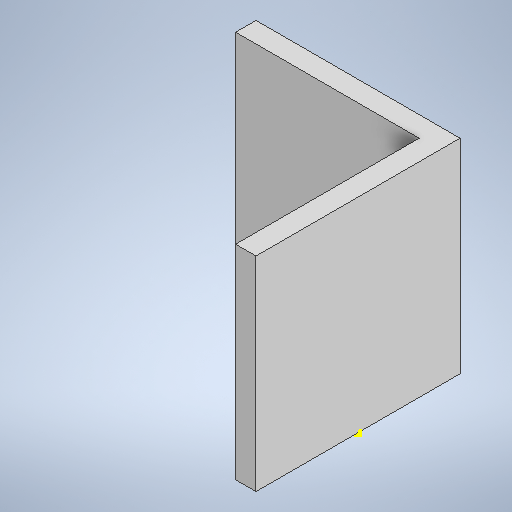
# Autodesk Inventor part: Soccer Goal Split
Saved by Autodesk Inventor 2026.1 (Build 301233000, 233)
## iProperties
Created: 2026-01-06
Part Number: Soccer Goal Split
Material: Generic
Document SubType Name: Modeling
Designer: User
Density: 1 g/cm^3
Appearance: Default
Author: User
Autodesk Inventor part; units mm, degrees
ref_plane "YZ Plane" through (0, 0, 0) normal (1, 0, 0) x (0, 1, 0)
ref_plane "XZ Plane" through (0, 0, 0) normal (0, 1, 0) x (-1, 0, 0)
ref_plane "XY Plane" through (0, 0, 0) normal (0, 0, 1) x (1, 0, 0)
sketch "Sketch1" plane through (0, 0, 0) normal (0, 1, 0) x (-1, 0, 0)
  line L0 (400, -50) -> (400, 50)
  line L1 (400, 50) -> (390, 50)
  line L2 (390, 50) -> (390, -40)
  line L3 (390, -40) -> (300, -40)
  line L4 (300, -40) -> (300, -50)
  line L5 (300, -50) -> (400, -50)
  line L6 (250, -50) -> (250, -40)
  line L7 (250, -40) -> (150, -40)
  line L8 (150, -40) -> (150, -50)
  line L9 (150, -50) -> (250, -50)
  line L10 (100, -50) -> (100, -40)
  line L11 (100, -40) -> (10, -40)
  line L12 (10, -40) -> (10, 50)
  line L13 (10, 50) -> (0, 50)
  line L14 (0, 50) -> (0, -50)
  line L15 (0, -50) -> (100, -50)
  point P0 (0, 0)
  dimension "d0" = 100
  dimension "d1" = 100
  dimension "d2" = 10
  dimension "d3" = 10
  dimension "d4" = 100
  dimension "d5" = 100
  dimension "d6" = 100
  dimension "d7" = 10
  dimension "d8" = 10
  dimension "d9" = 50
  dimension "d10" = 50
  dimension "d11" = 400
  dimension "d12" = 50
  dimension "d13" = 50
  constraints: 32 end point, 13 perpendicular, 4 point on line, 2 vertical
  measures "d0" distance of L0.start L0.end
  measures "d1" distance of L4.end L0.start
  measures "d2" distance of L0.end L1.end
  measures "d3" distance of L3.end L4.end
  measures "d4" distance of L8.end L6.start
  measures "d5" distance of L14.end L10.start
  measures "d6" distance of L13.end L14.end
  measures "d7" distance of L12.end L13.end
  measures "d8" distance of L10.start L10.end
  measures "d9" distance from line of L6.end L4
  measures "d10" distance between parallel lines of L10 L8
  measures "d11" distance from line of L0 point (0, 0)
  measures "d12" distance from line of point (0, 0) L5
  measures "d13" distance from line of point (0, 0) L13
extrude "Extrusion1" add sketch "Sketch1" along normal blind 100
sketch "Sketch2" plane through (0, 0, 0) normal (1, 0, 0) x (0, 1, 0)
  point P0 (0, 0)
sketch "Sketch3" plane through (0, 0, 50) normal (1, 0, 0) x (0, 0, -1)
  line L0 (92.5, 80) -> (97.5, 80)
  line L1 (97.5, 80) -> (97.5, 75)
  line L2 (97.5, 75) -> (92.5, 75)
  line L3 (92.5, 75) -> (92.5, 80)
  line L4 (97.5, 20) -> (92.5, 20)
  line L5 (92.5, 20) -> (92.5, 25)
  line L6 (92.5, 25) -> (97.5, 25)
  line L7 (97.5, 25) -> (97.5, 20)
  line L8 (0, 100) -> (100, 100) projected
  line L9 (100, 0) -> (100, 100) projected
  line L10 (0, 0) -> (100, 0) projected
  line L11 (92.5, 52.5) -> (97.5, 52.5)
  line L12 (97.5, 52.5) -> (97.5, 47.5)
  line L13 (97.5, 47.5) -> (92.5, 47.5)
  line L14 (92.5, 47.5) -> (92.5, 52.5)
  point P0 (50, 0)
  dimension "d16" = 20
  dimension "d17" = 5
  dimension "d18" = 5
  dimension "d19" = 2.5
  dimension "d20" = 20
  dimension "d21" = 5
  dimension "d22" = 5
  dimension "d24" = 7.5
  dimension "d25" = 5
  dimension "d26" = 5
  dimension "d27" = 2.5
  dimension "d28" = 22.5
  constraints: 24 end point, 6 parallel, 3 horizontal, 3 perpendicular
  measures "d16" distance between parallel lines of L8 L0
  measures "d17" distance of L1.end L2.end
  measures "d18" distance of L0.end L1.end
  measures "d19" distance between parallel lines of L9 L1
  measures "d20" distance between parallel lines of L10 L4
  measures "d21" distance of L6.end L4.start
  measures "d22" distance of L5.end L6.end
  measures "d24" distance between parallel lines of L9 L5
  measures "d25" distance of L13.end L11.start
  measures "d26" distance of L11.start L11.end
  measures "d27" distance between parallel lines of L9 L12
  measures "d28" distance between parallel lines of L2 L11
extrude "Extrusion2" cut sketch "Sketch3" against normal blind 320
sketch "Sketch4" plane through (0, 0, 50) normal (1, 0, 0) x (0, 0, -1)
  line L0 (97.5, 75) -> (92.5, 75) projected
  line L1 (97.5, 80) -> (97.5, 75) projected
  line L2 (92.5, 80) -> (97.5, 80) projected
  line L3 (92.5, 75) -> (92.5, 80) projected
  line L4 (97.5, 47.5) -> (92.5, 47.5) projected
  line L5 (97.5, 52.5) -> (97.5, 47.5) projected
  line L6 (92.5, 52.5) -> (97.5, 52.5) projected
  line L7 (92.5, 47.5) -> (92.5, 52.5) projected
  line L8 (92.5, 25) -> (97.5, 25) projected
  line L9 (92.5, 20) -> (92.5, 25) projected
  line L10 (97.5, 20) -> (92.5, 20) projected
  line L11 (97.5, 25) -> (97.5, 20) projected
  line L12 (92.5, 80) -> (97.5, 80)
  line L13 (97.5, 80) -> (97.5, 75)
  line L14 (97.5, 75) -> (92.5, 75)
  line L15 (92.5, 75) -> (92.5, 80)
  line L16 (92.5, 52.5) -> (97.5, 52.5)
  line L17 (97.5, 52.5) -> (97.5, 47.5)
  line L18 (97.5, 47.5) -> (92.5, 47.5)
  line L19 (92.5, 47.5) -> (92.5, 52.5)
  line L20 (92.5, 25) -> (97.5, 25)
  line L21 (97.5, 25) -> (97.5, 20)
  line L22 (97.5, 20) -> (92.5, 20)
  line L23 (92.5, 20) -> (92.5, 25)
  point P0 (50, 0)
  constraints: 24 end point, 6 parallel, 3 horizontal, 3 perpendicular
extrude "Extrusion3" add sketch "Sketch4" against normal blind 80
sketch "Sketch6" plane through (-250, 0, -40) normal (0, 0, 1) x (1, 0, 0)
  line L0 (-50, 80) -> (-50, 75) projected
  line L1 (-50, 80) -> (-70, 80) projected
  line L2 (-70, 80) -> (-70, 75) projected
  line L3 (-50, 75) -> (-70, 75) projected
  line L4 (-50, 52.5) -> (-50, 47.5) projected
  line L5 (-50, 52.5) -> (-70, 52.5) projected
  line L6 (-70, 52.5) -> (-70, 47.5) projected
  line L7 (-50, 47.5) -> (-70, 47.5) projected
  line L8 (-50, 25) -> (-50, 20) projected
  line L9 (-50, 25) -> (-70, 25) projected
  line L10 (-70, 25) -> (-70, 20) projected
  line L11 (-50, 20) -> (-70, 20) projected
  line L12 (0, 75) -> (0, 80) projected
  line L13 (100, 75) -> (0, 75) projected
  line L14 (100, 80) -> (100, 75) projected
  line L15 (100, 80) -> (0, 80) projected
  line L16 (0, 47.5) -> (0, 52.5) projected
  line L17 (100, 47.5) -> (0, 47.5) projected
  line L18 (100, 52.5) -> (100, 47.5) projected
  line L19 (100, 52.5) -> (0, 52.5) projected
  line L20 (0, 20) -> (0, 25) projected
  line L21 (100, 20) -> (0, 20) projected
  line L22 (100, 25) -> (100, 20) projected
  line L23 (100, 25) -> (0, 25) projected
  line L24 (170, 75) -> (170, 80) projected
  line L25 (170, 80) -> (150, 80) projected
  line L26 (150, 75) -> (150, 80) projected
  line L27 (170, 75) -> (150, 75) projected
  line L28 (170, 47.5) -> (170, 52.5) projected
  line L29 (170, 52.5) -> (150, 52.5) projected
  line L30 (150, 47.5) -> (150, 52.5) projected
  line L31 (170, 47.5) -> (150, 47.5) projected
  line L32 (170, 20) -> (170, 25) projected
  line L33 (170, 25) -> (150, 25) projected
  line L34 (150, 20) -> (150, 25) projected
  line L35 (170, 20) -> (150, 20) projected
  line L36 (-70, 80) -> (-60, 80)
  line L37 (-60, 80) -> (-60, 20)
  line L38 (-60, 20) -> (-70, 20)
  line L39 (-70, 20) -> (-70, 80)
  line L40 (10, 80) -> (90, 80)
  line L41 (90, 80) -> (90, 20)
  line L42 (90, 20) -> (10, 20)
  line L43 (10, 20) -> (10, 80)
  line L44 (160, 80) -> (170, 80)
  line L45 (170, 80) -> (170, 20)
  line L46 (170, 20) -> (160, 20)
  line L47 (160, 20) -> (160, 80)
  line L48 (0, 0) -> (0, 100) projected
  line L49 (100, 0) -> (100, 100) projected
  line L50 (10, 25) -> (90, 25)
  line L51 (90, 25) -> (90, 20)
  line L52 (90, 20) -> (10, 20)
  line L53 (10, 20) -> (10, 25)
  point P0 (250, 0)
  point P1 (160, 25)
  point P2 (160, 20)
  point P3 (160, 52.5)
  point P4 (160, 47.5)
  point P5 (160, 75)
  point P6 (10, 75)
  point P7 (90, 75)
  point P8 (90, 80)
  point P9 (10, 52.5)
  point P10 (10, 47.5)
  point P11 (90, 47.5)
  point P12 (90, 52.5)
  point P13 (10, 25)
  point P14 (10, 20)
  point P15 (-60, 25)
  point P16 (-60, 47.5)
  point P17 (-60, 52.5)
  point P18 (-60, 75)
  point P19 (90, 25)
  point P20 (90, 25)
  dimension "d33" = 10
  dimension "d34" = 10
  constraints: 32 end point, 8 parallel, 4 horizontal, 4 perpendicular, 4 point on line, 2 midpoint
  measures "d33" distance between parallel lines of L48 L43
  measures "d34" distance between parallel lines of L49 L41
extrude "Extrusion4" add sketch "Sketch6" against normal blind 10 contours L37 L3 L2 L1 | L37 L5 L39 L3 | L37 L7 L6 L5 | L37 L9 L39 L7 | L37 L11 L10 L9 | L43 L15 L41 L13 | L19 L41 L17 L43 | L23 L41 L21 L43 | L27 L47 L25 L24 | L45 L29 L47 L27 | L28 L31 L47 L29 | L45 L33 L47 L31 | L32 L35 L47 L33
sketch "Sketch8" plane through (0, 100, 0) normal (0, 1, 0) x (1, 0, 0)
  line L0 (-300, 50) -> (-400, 50) projected
  line L1 (-400, 50) -> (-400, -50) projected
  line L2 (-150, 40) -> (-150, 50) projected
  line L3 (-400, 50) -> (-150, 50)
  line L4 (-150, 50) -> (-150, -50)
  line L5 (-150, -50) -> (-400, -50)
  line L6 (-400, -50) -> (-400, 50)
  point P0 (0, 0)
  dimension "d44" = 250
  dimension "d45" = 100
  constraints: 8 end point, 2 parallel, 1 horizontal, 1 perpendicular
  measures "d44" distance of L4.end L5.end
  measures "d45" distance of L3.end L4.end
extrude "Extrusion6" cut sketch "Sketch8" against normal through all
body "Solid1"
